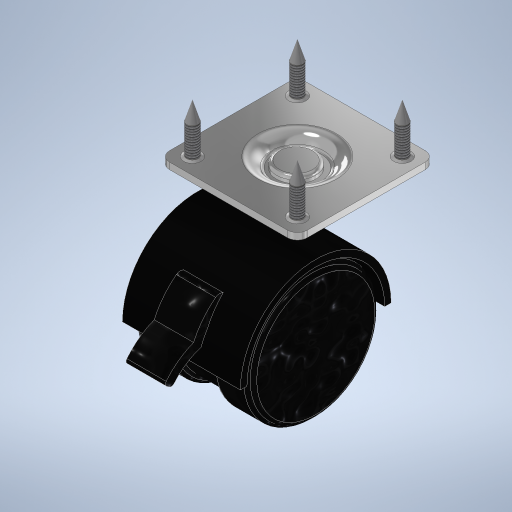
# Autodesk Inventor part: Wheel set with brake D40 H55
Saved by Autodesk Inventor 2024 (Build 280153000, 153)
## iProperties
Category: Support and legs
Created: 2007-05-24
Part Number: Wheel set with brake D40 H55
Material: ABS Plastic
Document SubType Name: Modeling
Designer: G.K.
Description: Wheel set
Authority: Design by UAB Čeli APS
Mass: 28.9774 g
Surface Area: 246.652 cm^2
Volume: 27.3372 cm^3
Density: 1.06 g/cm^3
Appearance: Black
Mase: 0.02897742
Author: G.K.
Title: Wheel set
Subject: Rollers
Keywords: wheel, set, rubber, brake, D40, D50, H55, H65
Comments: wheel, set, rubber, brake, D40, D50, H55, H65, Wheel set
Revision Number: 1
Autodesk Inventor part; units mm, degrees
ref_plane "YZ Plane" through (0, 0, 0) normal (1, 0, 0) x (0, 1, 0)
sketch "Sketch2" plane through (0, 0, 0) normal (0, 1, 0) x (-1, 0, 0)
  line L0 (0, -4) -> (0, 24) projected
  line L1 (-20.4, 0) -> (3.4, 0) projected
  line L2 (-17, 20) -> (-6.5, 20)
  line L3 (-6.5, 20) -> (-6.5, 0)
  line L4 (-7.5, 0) -> (-7.5, 19)
  line L5 (-7.5, 19) -> (-17, 19)
  line L6 (-17, 19) -> (-17, 20)
  point P0 (0, 0)
  dimension "d2" = 1
  dimension "d3" = 1
  dimension "d4" = 6.5
  dimension "d7" = 40
  dimension "d8" = 10.5
  constraints: 10 end point, 3 parallel, 2 perpendicular, 2 point on line
  measures "d2" distance between parallel lines of L5 L2
  measures "d3" distance between parallel lines of L3 L4
  measures "d4" distance between parallel lines of L3 L0
  measures "d7" diameter of L2 L1
  measures "d8" distance between parallel lines of L6 L3
revolve "Revolution1" add sketch "Sketch2" angle 360 about axis through (0, 0, 0) along (-1, 0, 0)
sketch "Sketch3" plane through (0, 0, 0) normal (0, 1, 0) x (-1, 0, 0)
  line L0 (-21.6, 0) -> (3.6, 0) projected
  line L1 (-16, 0) -> (-18, 0)
  line L2 (-18, 0) -> (-18, 19)
  line L3 (-18, 19) -> (-16, 19)
  line L4 (-16, 19) -> (-16, 0)
  line L5 (-17, -20) -> (-17, 20) projected
  point P0 (0, 0)
  dimension "d11" = 2
  dimension "d12" = 1
  dimension "d13" = 38
  constraints: 8 end point, 2 parallel, 1 horizontal, 1 perpendicular, 1 point on line
  measures "d11" distance between parallel lines of L4 L2
  measures "d12" distance between parallel lines of L5 L2
  measures "d13" diameter of L3 L0
revolve "Revolution2" add sketch "Sketch3" angle 360 about axis through (0, 0, 0) along (-1, 0, 0)
fillet "Fillet1" radius 1 3 edges at (6.5, 0, -20) (17, 0, -20) (18, 0, -19)
mirror "Mirror1" about plane through (0, 0, 0) normal (1, 0, 0) of "Revolution1", "Revolution2", "Fillet1"
sketch "Sketch4" plane through (0, 0, 0) normal (0, 1, 0) x (-1, 0, 0)
  line L0 (0, -3.6) -> (0, 21.6) projected
  line L1 (-6, 18) -> (6, 18)
  line L2 (6, 18) -> (6, 0)
  line L3 (6, 0) -> (-6, 0)
  line L4 (-6, 0) -> (-6, 18)
  line L5 (-8.4, 0) -> (8.4, 0) projected
  point P0 (0, 0)
  dimension "d16" = 36
  dimension "d17" = 12
  constraints: 8 end point, 2 parallel, 1 collinear, 1 horizontal, 1 perpendicular, 1 other
  measures "d16" diameter of L1 L5
  measures "d17" distance between parallel lines of L2 L4
revolve "Revolution3" add sketch "Sketch4" angle 360 about axis through (0, 0, 0) along (-1, 0, 0)
sketch "Sketch5" plane through (0, 0, 0) normal (1, 0, 0) x (0, 1, 0)
  arc A0 (21, 0) -> (-21, 0) centre (0, 0) ccw
  arc A1 (23, 0) -> (-23, 0) centre (0, 0) ccw
  line L0 (-32.2, 0) -> (32.2, 0) projected
  dimension "d19" = 42
  dimension "d20" = 2
  constraints: 4 point on circle, 4 point on line, 2 centre point, 1 coincident
  measures "d19" diameter of A0
  measures "d20" radial gap between concentric circles of A1 A0
extrude "Extrusion1" add sketch "Sketch5" against normal up to surface (36 mm away) from surface at 18 contours A0 L0 A1
sketch "Sketch6" plane through (0, 0, 0) normal (1, 0, 0) x (0, 1, 0)
  line L0 (12, 28) -> (18, 28)
  line L1 (18, 28) -> (18, 0)
  line L2 (18, 0) -> (12, 0)
  line L3 (12, 0) -> (12, 28)
  line L4 (0, 37.6) -> (0, -29.6) projected
  circle A0 centre (0, 0) radius 20 projected
  dimension "d23" = 12
  dimension "d24" = 6
  dimension "d25" = 28
  constraints: 8 end point, 2 parallel, 1 horizontal, 1 perpendicular, 1 point on line
  measures "d23" distance between parallel lines of L3 L4
  measures "d24" distance between parallel lines of L1 L3
  measures "d25" distance from line of A0.centre L0
revolve "Revolution4" add sketch "Sketch6" angle 360 about axis through (0, 12, 0) along (0, 0, 1) contours L0 L1 A0 L3 | A0 L1 L2 L3
sketch "Sketch7" plane through (0, 0, 0) normal (0, 1, 0) x (-1, 0, 0)
  line L0 (-12.6, 0) -> (12.6, 0) projected
  line L1 (9, 0) -> (9, 7)
  line L2 (9, 7) -> (7.7, 7)
  line L3 (7.7, 7) -> (7.7, 5)
  line L4 (7.7, 5) -> (-7.7, 5)
  line L5 (-7.7, 5) -> (-7.7, 7)
  line L6 (-7.7, 7) -> (-9, 7)
  line L7 (-9, 7) -> (-9, 0)
  line L8 (7.5, -20) -> (7.5, 20) projected
  line L9 (-7.5, -19) -> (-7.5, 19) projected
  line L10 (0, -28) -> (0, 28) projected
  point P0 (0, 0)
  dimension "d27" = 0.2
  dimension "d28" = 0.2
  dimension "d29" = 14
  dimension "d30" = 10
  dimension "d31" = 18
  constraints: 14 end point, 3 parallel, 3 perpendicular, 2 collinear, 2 point on line, 1 other
  measures "d27" distance between parallel lines of L8 L3
  measures "d28" distance between parallel lines of L5 L9
  measures "d29" diameter of L2 L0
  measures "d30" diameter of L4 L0
  measures "d31" distance between parallel lines of L7 L1
revolve "Revolution5" add sketch "Sketch7" angle 360 about axis through (0, 0, 0) along (-1, 0, 0)
sketch "Sketch8" plane through (0, 0, 0) normal (1, 0, 0) x (0, 1, 0)
  arc A0 (-18.5196, 16.2263) -> (-25.2655, 7.6843) centre (-5.1638, -1.2558) ccw
  arc A1 (-25.2655, 7.6843) -> (-33.6302, 1.6) centre (-18.0834, -10.9817) ccw
  arc A2 (-23, 5.2918) -> (-31.2298, -0.2034) centre (-18.0834, -10.9817) ccw
  arc A3 (-15, 15) -> (-23, 5.2918) centre (-5.1638, -1.2558) ccw
  line L0 (-33.3894, 0.127) -> (-32.5397, -0.4132)
  line L1 (-15.7727, 15.9218) -> (-15, 15)
  arc A4 (-15.7727, 15.9218) -> (-18.5196, 16.2263) centre (-17.3055, 14.637) ccw
  arc A5 (-33.6302, 1.6) -> (-33.3894, 0.127) centre (-32.8528, 0.9709) ccw
  arc A6 (-32.5397, -0.4132) -> (-31.2298, -0.2034) centre (-32.0031, 0.4306) ccw
  point P0 (0, 0)
  dimension "d42" = 3
  dimension "d43" = 17
  dimension "d44" = 20
  dimension "d45" = 19
  dimension "d46" = 22
  dimension "d47" = 2
  dimension "d48" = 1
  dimension "d49" = 15
  dimension "d50" = 15
  dimension "d51" = 23
  constraints: 14 point on circle, 7 centre point, 6 tangent, 4 end point, 1 equal radius, 1 other
  measures "d42" radial gap between concentric circles of A2 A1
  measures "d43" radius of A2
  measures "d44" radius of A1
  measures "d45" radius of A3
  measures "d46" radius of A0
  measures "d47" radius of A4
  measures "d48" radius of A5
  measures "d49" horizontal distance of L1.end point (0, 0)
  measures "d50" horizontal distance of L1.end point (0, 0)
  measures "d51" horizontal distance of point (0, 0) A2.start
extrude "Extrusion2" add sketch "Sketch8" along normal mid plane 12
hole "Hole1" at (0, 12, 28) direction (0, 0, -1) diameter 8 depth 35 tip angle 118
sketch "Sketch9" plane through (0, 0, 0) normal (1, 0, 0) x (0, 1, 0)
  line L0 (8, 28) -> (16, 28) projected
  line L1 (12, 47.749) -> (12, -7)
  line L2 (12, -13) -> (12, 43)
  line L3 (12, 34.2) -> (6, 34.2)
  line L4 (6, 34.2) -> (6, 32.2)
  line L5 (6, 32.2) -> (8, 32.2)
  line L6 (8, 32.2) -> (8, 1)
  line L7 (8, 1) -> (8.5, 1)
  line L8 (8.5, 1) -> (8.5, -3)
  line L9 (8.5, -3) -> (8, -3)
  line L10 (8, -3) -> (8, -5)
  line L11 (8, -5) -> (12, -5)
  line L12 (19.2029, 32) -> (4.7971, 32)
  line L13 (23.9857, 35) -> (0.0143, 35)
  line L14 (6, 28) -> (18, 28) projected
  point P0 (0, 0)
  point P1 (12, 28)
  point P2 (12, 33)
  dimension "d54" = 7
  dimension "d55" = 8
  dimension "d56" = 12
  dimension "d57" = 2
  dimension "d58" = 0.2
  dimension "d59" = 4
  dimension "d60" = 2
  dimension "d61" = 40
  dimension "d62" = 35
  dimension "d120" = 4
  constraints: 26 end point, 6 parallel, 4 perpendicular, 2 point on line, 1 collinear, 1 midpoint, 1 vertical
  measures "d54" diameter of L8 L2
  measures "d55" diameter of L6 L2
  measures "d56" diameter of L4 L2
  measures "d57" distance between parallel lines of L5 L3
  measures "d58" distance between parallel lines of L12 L5
  measures "d59" distance from line of L8.end L7
  measures "d60" distance between parallel lines of L11 L9
  measures "d61" distance between parallel lines of L13 L11
  measures "d62" distance of L1.end point (12, 28)
  measures "d120" distance between parallel lines of L14 L12
revolve "Revolution6" add sketch "Sketch9" angle 360 about axis through (0, 12, -13) along (0, 0, 1) separate body
ref_plane "Work Plane1" through (0, 12, 35) normal (0, 0, 1) x (1, 0, 0)
sketch "Sketch10" plane through (0, 0, 0) normal (1, 0, 0) x (0, 1, 0)
  line L0 (-45.2234, 35) -> (34.3706, 35) construction
  line L1 (12.3844, 39.1999) -> (12.3844, 30.8234)
  line L2 (-17.6156, 35) -> (-17.6156, 33)
  line L3 (-17.6156, 33) -> (0.8019, 33)
  line L4 (5.3844, 30) -> (12.3844, 30)
  line L5 (12.3844, 32) -> (5.1816, 32)
  line L6 (0.3987, 35) -> (-17.6156, 35)
  line L7 (12.3844, 32) -> (12.3844, 30)
  line L8 (4.3844, 32.5) -> (4.3844, 31.93)
  line L9 (2.3844, 33) -> (2.3844, 33)
  arc A0 (2.6349, 31.8) -> (5.3844, 30) centre (5.3844, 33) ccw
  arc A1 (2.6349, 31.8) -> (0.8019, 33) centre (0.8019, 31) ccw
  arc A2 (4.3844, 32.5) -> (0.3987, 35) centre (0.3987, 30.5728) ccw
  arc A3 (4.3844, 32.5) -> (5.1816, 32) centre (5.1816, 32.8854) ccw
  line L10 (18, 34.2) -> (6, 34.2) projected
  point P0 (0, 0)
  point P1 (6, 34.2)
  point P2 (12.3844, 37.2)
  dimension "d65" = 2
  dimension "d66" = 2
  dimension "d67" = 60
  dimension "d68" = 2
  dimension "d69" = 3
  dimension "d70" = 16
  dimension "d71" = 5
  dimension "d72" = 2
  dimension "d73" = 0.8854
  dimension "d74" = 4.4272
  constraints: 18 end point, 9 point on circle, 7 tangent, 5 parallel, 4 centre point, 2 collinear, 2 point on line, 1 perpendicular, 3 other
  measures "d65" distance between parallel lines of L3 L6
  measures "d66" distance between parallel lines of L4 L5
  measures "d67" diameter of L2 L1
  measures "d68" distance between parallel lines of L9 L8
  measures "d69" radius of A0
  measures "d70" diameter of L8 L1
  measures "d71" distance between parallel lines of L6 L4
  measures "d72" radius of A1
  measures "d73" radius of A3
  measures "d74" radius of A2
revolve "Revolution7" add sketch "Sketch10" angle 360 about axis through (0, 12.3844, 39.1999) along (0, 0, -1) separate body
sketch "Sketch11" plane through (0, 12.3844, 35) normal (0, 0, 1) x (1, 0, 0)
  circle A0 centre (0, 0) radius 30 projected
  circle A1 centre (0, 0) radius 11.9857 projected
  line L0 (-21, 21) -> (21, 21)
  line L1 (21, 21) -> (21, -21)
  line L2 (21, -21) -> (-21, -21)
  line L3 (-21, -21) -> (-21, 21)
  line L4 (-21, 21) -> (21, -21) construction
  line L5 (21, 21) -> (-21, -21) construction
  point P0 (0, -12.3844)
  dimension "d76" = 42
  dimension "d77" = 42
  constraints: 12 end point, 2 midpoint, 2 parallel, 1 horizontal, 1 perpendicular
  measures "d76" distance of L1.end L2.end
  measures "d77" distance of L0.end L1.end
extrude "Extrusion3" cut sketch "Sketch11" against normal through all contours A0 bodies 3
fillet "Fillet3" radius 3 4 edges at (-21, -8.6156, 34) (21, -8.6156, 34) (21, 33.3844, 34) (-21, 33.3844, 34)
fillet "Fillet3" radius 1 1 edges at (0, 18, 34.2)
sketch "Sketch12" plane through (-18, -8.6156, 35) normal (0, 0, 1) x (1, 0, 0)
  circle A0 centre (18, 21) radius 11.9857 projected
  line L0 (2, 5) -> (34, 5)
  line L1 (34, 5) -> (34, 37)
  line L2 (34, 37) -> (2, 37)
  line L3 (2, 37) -> (2, 5)
  line L4 (2, 5) -> (34, 37) construction
  line L5 (34, 5) -> (2, 37) construction
  point P0 (18, 8.6156)
  dimension "d82" = 32
  dimension "d83" = 32
  constraints: 12 end point, 2 midpoint, 2 parallel, 1 horizontal, 1 perpendicular
  measures "d82" distance of L2.end L1.end
  measures "d83" distance of L1.end L0.end
hole "Hole2" at (16, 28.3844, 35) at (-16, 28.3844, 35) at (16, -3.6156, 35) at (-16, -3.6156, 35) direction (0, 0, -1) diameter 5.3 end through all bodies 3
ref_plane "Work Plane2" through (16, -3.6156, -24.607) normal (1, 0, 0) x (0, 0, 1)
sketch "Sketch13" plane through (16, -3.6156, -24.607) normal (1, 0, 0) x (0, 0, 1)
  line L0 (57.607, -2.65) -> (57.607, 2.65) projected
  line L1 (57.607, 4.2) -> (57.607, -0.7) construction
  line L2 (54.207, 0) -> (78.007, 0)
  line L3 (57.607, 0) -> (57.607, 3.5)
  line L4 (57.607, 3.5) -> (58.107, 3.5)
  line L5 (58.107, 3.5) -> (59.857, 1.75)
  line L6 (59.857, 1.75) -> (68.8831, 1.75)
  line L7 (68.8831, 1.75) -> (74.607, 0)
  point P0 (24.607, -3.6156)
  dimension "d92" = 3.5
  dimension "d93" = 7
  dimension "d94" = 0.5
  dimension "d95" = 45
  dimension "d96" = 17
  dimension "d97" = 17
  dimension "d98" = 9.026
  constraints: 14 end point, 2 perpendicular, 2 point on line, 1 collinear, 1 midpoint, 1 parallel, 1 other
  measures "d92" diameter of L6 L2
  measures "d93" diameter of L4 L2
  measures "d94" distance from line of L4.end L3
  measures "d95" angle of L5 L3
  measures "d96" distance from line of L7.end L3
  measures "d97" angle of L7 L2
  measures "d98" distance of L5.end L6.end
revolve "Revolution8" add sketch "Sketch13" angle 360 about axis through (16, -3.6156, 29.6) along (0, 0, 1) separate body
sketch "Sketch14" plane through (16, -3.6156, -24.607) normal (1, 0, 0) x (0, 0, 1)
  line L0 (59.767, 0) -> (57.247, 0)
  line L1 (59.407, 0) -> (59.407, -0.9896)
  line L2 (59.407, -0.9896) -> (57.607, -2.5)
  line L3 (57.607, -2.5) -> (57.607, 0)
  line L4 (57.607, -3.5) -> (57.607, 3.5)
  line L5 (57.607, -2.65) -> (57.607, 2.65) projected
  point P0 (24.607, -3.6156)
  point P1 (57.607, 0)
  dimension "d100" = 40
  dimension "d101" = 1.8
  dimension "d102" = 2.5
  constraints: 10 end point, 2 perpendicular, 2 point on line, 1 collinear, 1 midpoint
  measures "d100" angle of L2 L0
  measures "d101" distance between parallel lines of L1 L3
  measures "d102" distance from line of L0 L2.end
extrude "Extrusion4" cut sketch "Sketch14" along normal mid plane 1 bodies 4
pattern_circular "Circular Pattern1" count 4 over 360 about axis through (16, -3.6156, 39.763) along (0, 0, 1) of "Extrusion4" bodies 4
thread "Thread1" size "M4x0.7" class "6g" standard "ANSI Metric M Profile" full length
pattern_linear "Rectangular Pattern1" count 2 spacing 32 along (-1, 0, 0) count 2 spacing 32 along (0, 1, 0) bodies 4
equation "\"d7\" = Wheel_dia"
equation "\"Wheel_dia\" = 40"
equation "\"Wheel_H\" = 55"
